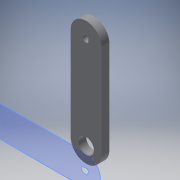
# Autodesk Inventor part: Part5
Saved by Autodesk Inventor 2016 (Build 200138000, 138)
## iProperties
Created: 2017-09-19
Part Number: Part5
Material: Generic
Document SubType Name: Modeling
Designer: student
Density: 1 g/cm^3
Appearance: Default
Author: student
Autodesk Inventor part; units mm, degrees
ref_plane "YZ Plane" through (0, 0, 0) normal (1, 0, 0) x (0, 1, 0)
ref_plane "XZ Plane" through (0, 0, 0) normal (0, 1, 0) x (-1, 0, 0)
ref_plane "XY Plane" through (0, 0, 0) normal (0, 0, 1) x (1, 0, 0)
sketch "Sketch1" plane through (0, 0, 0) normal (0, 0, 1) x (1, 0, 0)
  circle A0 centre (49.1868, 0) radius 3.175
  arc A1 (50.1181, 39.1289) -> (50.1181, 37.0464) centre (49.1868, 38.0877) ccw
  line L0 (49.1868, 38.0877) -> (49.1868, 0) construction
  line L1 (42.8368, 38.0877) -> (42.8368, 0)
  line L2 (55.5368, 0) -> (55.5368, 38.0877)
  arc A2 (55.5368, 38.0877) -> (42.8368, 38.0877) centre (49.1868, 38.0877) ccw
  arc A3 (42.8368, 0) -> (55.5368, 0) centre (49.1868, 0) ccw
  line L3 (47.7898, 38.0877) -> (50.3298, 38.0877) construction
  line L4 (50.1181, 37.0464) -> (50.1181, 39.1289)
  point P0 (49.1868, 19.0438)
  dimension "d0" = 12.7
  dimension "d3" = 2.794
  dimension "d4" = 2.54
  constraints: 12 end point, 7 point on circle, 4 centre point, 4 tangent, 2 vertical, 1 horizontal, 1 midpoint, 1 parallel
  measures "d0" diameter of A3
  measures "d3" diameter of A1
  measures "d4" distance of L3.start L3.end
extrude "Extrusion1" add sketch "Sketch1" along normal blind 3.175
body "Solid1"
